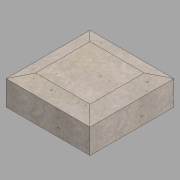
# Autodesk Inventor part: Full_Cap_1
Saved by Autodesk Inventor 2022.1 (Build 261234020, 234B)
## iProperties
Created: 2021-12-03
Part Number: Full_Cap_1
Material: Limestone
Document SubType Name: Modeling
Designer: awelt
Density: 2.6 g/cm^3
Appearance: Kasota Gray
Mass: 560359 g
Surface Area: 23924.8 cm^2
Volume: 215523 cm^3
Author: awelt
Autodesk Inventor part; units mm, degrees
ref_plane "YZ Plane" through (0, 0, 0) normal (1, 0, 0) x (0, 1, 0)
ref_plane "XZ Plane" through (0, 0, 0) normal (0, 1, 0) x (-1, 0, 0)
ref_plane "XY Plane" through (0, 0, 0) normal (0, 0, 1) x (1, 0, 0)
sketch "Sketch1" plane through (0, 0, 0) normal (0, 1, 0) x (-1, 0, 0)
  line L0 (431.8, -431.8) -> (-431.8, -431.8)
  line L1 (-431.8, -431.8) -> (-431.8, 431.8)
  line L2 (-431.8, 431.8) -> (431.8, 431.8)
  line L3 (431.8, 431.8) -> (431.8, -431.8)
  line L4 (431.8, -431.8) -> (-431.8, 431.8) construction
  line L5 (-431.8, -431.8) -> (431.8, 431.8) construction
  point P0 (0, 0)
  dimension "d0" = 863.6
  dimension "d1" = 863.6
  constraints: 12 end point, 2 midpoint, 2 parallel, 1 horizontal, 1 perpendicular
  measures "d0" distance of L1.end L2.end
  measures "d1" distance of L0.end L1.end
extrude "Extrusion1" add sketch "Sketch1" along normal blind 304.8
sketch "Sketch2" plane through (431.8, 0, 431.8) normal (1, 0, 0) x (0, 0, -1)
  line L0 (0, 0) -> (0, 304.8) projected
  line L1 (0, 304.8) -> (863.6, 304.8) projected
  line L2 (0, 254) -> (152.4, 304.8)
  line L3 (152.4, 304.8) -> (0, 304.8)
  line L4 (0, 304.8) -> (0, 254)
  point P0 (431.8, 0)
  dimension "d4" = 152.4
  dimension "d5" = 50.8
  constraints: 6 end point, 2 point on line, 1 collinear, 1 perpendicular
  measures "d4" distance of L2.end L0.end
  measures "d5" distance of L2.start L0.end
sketch3d "3D Sketch1"
  line L0 (431.8, 304.8, 431.8) -> (-431.8, 304.8, 431.8)
  line L1 (-431.8, 304.8, 431.8) -> (-431.8, 304.8, -431.8)
  line L2 (-431.8, 304.8, -431.8) -> (431.8, 304.8, -431.8)
  line L3 (431.8, 304.8, -431.8) -> (431.8, 304.8, 431.8)
sweep "Sweep1" cut profiles "Sketch2" path "3D Sketch1"
body "Solid1"
